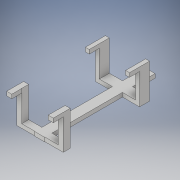
# Autodesk Inventor part: battery
Saved by Autodesk Inventor 2018.2 (Build 222227000, 227)
## iProperties
Created: 2018-03-29
Part Number: battery
Material: Generic
Document SubType Name: Modeling
Designer: MIABo
Density: 1 g/cm^3
Appearance: Default
Author: MIABo
Autodesk Inventor part; units mm, degrees
ref_plane "YZ Plane" through (0, 0, 0) normal (1, 0, 0) x (0, 1, 0)
ref_plane "XZ Plane" through (0, 0, 0) normal (0, 1, 0) x (-1, 0, 0)
ref_plane "XY Plane" through (0, 0, 0) normal (0, 0, 1) x (1, 0, 0)
sketch "Sketch1" plane through (0, 0, 0) normal (0, 1, 0) x (-1, 0, 0)
  line L0 (23.114, 69.469) -> (-23.114, 69.469)
  line L1 (-23.114, 69.469) -> (-23.114, -69.469)
  line L2 (-23.114, -69.469) -> (23.114, -69.469)
  line L3 (23.114, -69.469) -> (23.114, 69.469)
  line L4 (23.114, 69.469) -> (-23.114, -69.469) construction
  line L5 (-23.114, 69.469) -> (23.114, -69.469) construction
  line L6 (-29.464, 60.706) -> (29.464, 60.706)
  line L7 (29.464, 60.706) -> (29.464, 69.469)
  line L8 (29.464, 69.469) -> (-29.464, 69.469)
  line L9 (-29.464, 69.469) -> (-29.464, 60.706)
  line L10 (-29.464, 60.706) -> (29.464, 69.469) construction
  line L11 (29.464, 60.706) -> (-29.464, 69.469) construction
  line L12 (6.35, 69.85) -> (-6.35, 69.85)
  line L13 (-6.35, 69.85) -> (-6.35, -69.85)
  line L14 (-6.35, -69.85) -> (6.35, -69.85)
  line L15 (6.35, -69.85) -> (6.35, 69.85)
  line L16 (6.35, 69.85) -> (-6.35, -69.85) construction
  line L17 (-6.35, 69.85) -> (6.35, -69.85) construction
  point P0 (0, 0)
  point P1 (0, 65.0875)
  dimension "d0" = 46.228
  dimension "d1" = 138.938
  dimension "d2" = 58.928
  constraints: 36 end point, 6 midpoint, 6 parallel, 3 horizontal, 3 perpendicular
  measures "d0" distance of L2.end L1.end
  measures "d1" distance of L1.end L0.end
  measures "d2" distance of L8.end L7.end
sketch "Sketch2" plane through (0, 0, 0) normal (0, 1, 0) x (-1, 0, 0)
  line L0 (-9.525, 69.85) -> (-9.525, -28.575)
  line L1 (-38.1, -41.275) -> (38.1, -41.275)
  line L2 (38.1, -41.275) -> (38.1, -28.575)
  line L3 (38.1, -28.575) -> (-38.1, -28.575)
  line L4 (-38.1, -28.575) -> (-38.1, -41.275)
  line L5 (-38.1, -41.275) -> (38.1, -28.575) construction
  line L6 (38.1, -41.275) -> (-38.1, -28.575) construction
  point P0 (0, 0)
  point P1 (0, -34.925)
  dimension "d3" = 98.425
  dimension "d4" = 76.2
  constraints: 14 end point, 2 midpoint, 2 parallel, 1 horizontal, 1 perpendicular, 1 vertical
  measures "d3" distance of L0.start L0.end
  measures "d4" distance of L3.end L2.end
extrude "Extrusion1" add sketch "Sketch2" along normal blind 5.08
extrude "Extrusion2" add sketch "Sketch1" along normal blind 5.08 contours L3 L6 L15 L0 | L8 L7 L6 L3 | L15 L6 L13 L0 | L0 L13 L12 L15 | L13 L6 L1 L0 | L15 L2 L13 L6 | L1 L6 L9 L8 | L15 L14 L13 L2
sketch "Sketch3" plane through (0, 5.08, 0) normal (0, 1, 0) x (1, 0, 0)
  line L0 (-29.464, -60.706) -> (-29.464, -69.469) projected
  line L1 (-29.464, -69.469) -> (-6.35, -69.469) projected
  line L2 (-29.464, -60.706) -> (-23.114, -60.706)
  line L3 (-23.114, -60.706) -> (-23.114, -69.469)
  line L4 (-23.114, -69.469) -> (-29.464, -69.469)
  line L5 (-29.464, -69.469) -> (-29.464, -60.706)
  line L6 (29.464, -69.469) -> (29.464, -60.706) projected
  line L7 (6.35, -69.469) -> (29.464, -69.469) projected
  line L8 (29.464, -60.706) -> (23.114, -60.706)
  line L9 (23.114, -60.706) -> (23.114, -69.469)
  line L10 (23.114, -69.469) -> (29.464, -69.469)
  line L11 (29.464, -69.469) -> (29.464, -60.706)
  point P0 (0, 0)
  dimension "d9" = 6.35
  dimension "d10" = 6.35
  constraints: 16 end point, 4 parallel, 2 horizontal, 2 perpendicular, 2 point on line
  measures "d9" distance of L3.end L4.end
  measures "d10" distance of L10.end L9.end
extrude "Extrusion3" add sketch "Sketch3" along normal blind 38.735
sketch "Sketch4" plane through (0, 5.08, 0) normal (0, 1, 0) x (1, 0, 0)
  line L0 (-38.1, 41.275) -> (-38.1, 28.575) projected
  line L1 (-38.1, 28.575) -> (-6.35, 28.575) projected
  line L2 (-38.1, 41.275) -> (-22.987, 41.275)
  line L3 (-22.987, 41.275) -> (-22.987, 28.575)
  line L4 (-22.987, 28.575) -> (-38.1, 28.575)
  line L5 (-38.1, 28.575) -> (-38.1, 41.275)
  line L6 (38.1, 28.575) -> (38.1, 41.275) projected
  line L7 (6.35, 28.575) -> (38.1, 28.575) projected
  line L8 (38.1, 41.275) -> (22.987, 41.275)
  line L9 (22.987, 41.275) -> (22.987, 28.575)
  line L10 (22.987, 28.575) -> (38.1, 28.575)
  line L11 (38.1, 28.575) -> (38.1, 41.275)
  point P0 (0, 0)
  dimension "d13" = 15.113
  dimension "d14" = 15.113
  constraints: 16 end point, 4 parallel, 2 horizontal, 2 perpendicular, 2 point on line
  measures "d13" distance of L3.end L4.end
  measures "d14" distance of L10.end L9.end
extrude "Extrusion4" add sketch "Sketch4" along normal blind 38.735
sketch "Sketch5" plane through (-38.1, 0, -41.275) normal (-1, 0, 0) x (0, 0, 1)
  line L0 (-6.35, 53.975) -> (19.05, 53.975)
  line L1 (19.05, 53.975) -> (19.05, -3.175)
  line L2 (19.05, -3.175) -> (-6.35, -3.175)
  line L3 (-6.35, -3.175) -> (-6.35, 53.975)
  line L4 (-6.35, 53.975) -> (19.05, -3.175) construction
  line L5 (19.05, 53.975) -> (-6.35, -3.175) construction
  point P0 (41.275, 0)
  point P1 (6.35, 25.4)
  constraints: 12 end point, 2 midpoint, 2 parallel, 1 horizontal, 1 perpendicular
extrude "Extrusion5" cut sketch "Sketch5" against normal blind 10.16
sketch "Sketch6" plane through (6.35, 0, -28.575) normal (0, 0, 1) x (1, 0, 0)
  point P0 (-6.35, 0)
sketch "Sketch7" plane through (38.1, 0, -28.575) normal (1, 0, 0) x (0, 0, -1)
  line L0 (-1.5875, 49.2125) -> (17.4625, 49.2125)
  line L1 (17.4625, 49.2125) -> (17.4625, -4.7625)
  line L2 (17.4625, -4.7625) -> (-1.5875, -4.7625)
  line L3 (-1.5875, -4.7625) -> (-1.5875, 49.2125)
  line L4 (-1.5875, 49.2125) -> (17.4625, -4.7625) construction
  line L5 (17.4625, 49.2125) -> (-1.5875, -4.7625) construction
  point P0 (-28.575, 0)
  point P1 (7.9375, 22.225)
  constraints: 12 end point, 2 midpoint, 2 parallel, 1 horizontal, 1 perpendicular
extrude "Extrusion6" cut sketch "Sketch7" against normal blind 10.16
sketch "Sketch8" plane through (-29.464, 0, 69.469) normal (0, 0, 1) x (1, 0, 0)
  line L0 (0, 0) -> (0, 43.815) projected
  line L1 (6.477, 5.08) -> (6.477, 43.815) projected
  line L2 (0, 43.815) -> (6.477, 43.815)
  line L3 (6.477, 43.815) -> (6.477, 38.735)
  line L4 (6.477, 38.735) -> (0, 38.735)
  line L5 (0, 38.735) -> (0, 43.815)
  line L6 (58.928, 0) -> (58.928, 43.815) projected
  line L7 (52.451, 5.08) -> (52.451, 43.815) projected
  line L8 (58.928, 43.815) -> (52.451, 43.815)
  line L9 (52.451, 43.815) -> (52.451, 38.735)
  line L10 (52.451, 38.735) -> (58.928, 38.735)
  line L11 (58.928, 38.735) -> (58.928, 43.815)
  point P0 (29.464, 0)
  dimension "d21" = 5.08
  constraints: 16 end point, 4 parallel, 3 point on line, 2 horizontal, 2 perpendicular
  measures "d21" distance of L2.end L3.end
extrude "Extrusion7" add sketch "Sketch8" along normal blind 12.7
sketch "Sketch9" plane through (6.35, 0, -28.575) normal (0, 0, 1) x (1, 0, 0)
  line L0 (16.637, 5.08) -> (16.637, 43.815) projected
  line L1 (21.59, 43.815) -> (21.59, 0) projected
  line L2 (16.637, 43.815) -> (21.59, 43.815)
  line L3 (21.59, 43.815) -> (21.59, 38.735)
  line L4 (21.59, 38.735) -> (16.637, 38.735)
  line L5 (16.637, 38.735) -> (16.637, 43.815)
  line L6 (-34.29, 43.815) -> (-34.29, 0) projected
  line L7 (-29.337, 5.08) -> (-29.337, 43.815) projected
  line L8 (-34.29, 43.815) -> (-29.337, 43.815)
  line L9 (-29.337, 43.815) -> (-29.337, 38.735)
  line L10 (-29.337, 38.735) -> (-34.29, 38.735)
  line L11 (-34.29, 38.735) -> (-34.29, 43.815)
  point P0 (-6.35, 0)
  dimension "d24" = 5.08
  constraints: 16 end point, 4 parallel, 3 point on line, 2 horizontal, 2 perpendicular
  measures "d24" distance of L2.end L3.end
extrude "Extrusion8" add sketch "Sketch9" along normal blind 12.7
body "Solid1"
